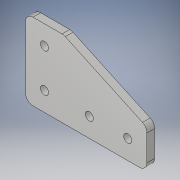
# Autodesk Inventor part: 上昇機構_固定具1
Saved by Autodesk Inventor 2019.4 (Build 234330000, 330)
## iProperties
Created: 2021-12-04
Part Number: 上昇機構_固定具1
Material: アルミニウム 6061
Document SubType Name: Modeling
Designer: 堀川皓史
Density: 2.7 g/cm^3
Appearance: アルミニウム - フラット
Author: 堀川皓史
Autodesk Inventor part; units mm, degrees
ref_plane "YZ Plane" through (0, 0, 0) normal (1, 0, 0) x (0, 1, 0)
ref_plane "XZ Plane" through (0, 0, 0) normal (0, 1, 0) x (-1, 0, 0)
ref_plane "XY Plane" through (0, 0, 0) normal (0, 0, 1) x (1, 0, 0)
sketch "スケッチ1" plane through (0, 0, 0) normal (0, 0, 1) x (1, 0, 0)
  circle A0 centre (0, 0) radius 1.6
  circle A1 centre (0, 15) radius 1.6
  circle A2 centre (17.5, 0) radius 1.6
  circle A3 centre (32.5, 0) radius 1.6
  line L0 (-7.5, 22.5) -> (7.5, 22.5)
  line L1 (7.5, 22.5) -> (40, 7.5)
  line L2 (-7.5, 22.5) -> (-7.5, -7.5)
  line L3 (-7.5, -7.5) -> (40, -7.5)
  line L4 (40, -7.5) -> (40, 7.5)
  dimension "d0" = 3.2
  dimension "d1" = 3.2
  dimension "d2" = 15
  dimension "d3" = 3.2
  dimension "d4" = 3.2
  dimension "d5" = 17.5
  dimension "d6" = 15
  dimension "d7" = 7.5
  dimension "d12" = 15
  dimension "d16" = 15
  dimension "d17" = 7.5
  dimension "d18" = 7.5
  dimension "d19" = 7.5
  constraints: 10 end point, 4 centre point, 2 horizontal, 2 horizontal alignment, 1 coincident, 1 perpendicular, 1 vertical, 1 vertical alignment
  measures "d0" diameter of A0
  measures "d1" diameter of A1
  measures "d2" distance of point (0, 0) A1.centre
  measures "d3" diameter of A2
  measures "d4" diameter of A3
  measures "d5" distance of A2.centre point (0, 0)
  measures "d6" distance of A3.centre A2.centre
  measures "d7" distance from line of A1.centre L0
  measures "d12" distance of L0.start L0.end
  measures "d16" distance of L3.end L1.end
  measures "d17" distance from line of L3 A3.centre
  measures "d18" distance from line of point (0, 0) L2
  measures "d19" distance from line of L4 A3.centre
extrude "押し出し1" add sketch "スケッチ1" along normal blind 3
fillet "フィレット1" radius 3 5 edges at (-7.5, 22.5, 1.5) (7.5, 22.5, 1.5) (40, 7.5, 1.5) (-7.5, -7.5, 1.5) (40, -7.5, 1.5)
